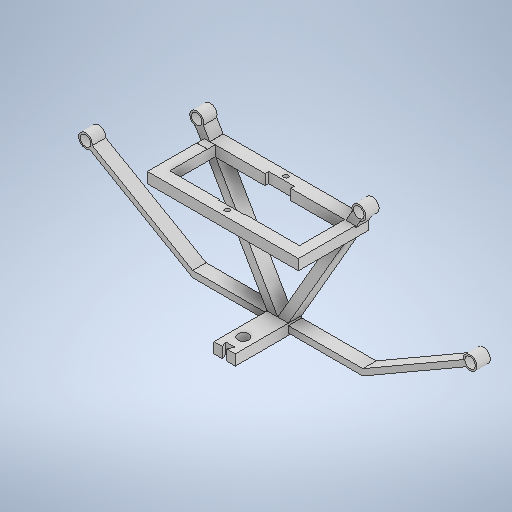
# Autodesk Inventor part: pelvis øvre del stor servo
Saved by Autodesk Inventor 2025.1 (Build 291241020, 241B)
## iProperties
Created: 2025-01-28
Part Number: pelvis øvre del stor servo
Material: Generic
Document SubType Name: Modeling
Designer: morte
Density: 1 g/cm^3
Appearance: Default
Author: morte
Autodesk Inventor part; units mm, degrees
ref_plane "XZ Plane" through (0, 0, 0) normal (0, 1, 0) x (-1, 0, 0)
ref_plane "XY Plane" through (0, 0, 0) normal (0, 0, 1) x (1, 0, 0)
sketch "Sketch1" plane through (0, 0, 0) normal (0, 0, 1) x (1, 0, 0)
  line L0 (5, -2.5) -> (-5, -2.5)
  line L1 (-5, -2.5) -> (-5, 2.5)
  line L2 (-5, 2.5) -> (5, 2.5)
  line L3 (5, 2.5) -> (5, -2.5)
  line L4 (5, -2.5) -> (-5, 2.5) construction
  line L5 (-5, -2.5) -> (5, 2.5) construction
  point P0 (0, 0)
  dimension "d0" = 10
  dimension "d1" = 5
  constraints: 12 end point, 2 midpoint, 2 parallel, 1 horizontal, 1 perpendicular
  measures "d0" distance of L1.end L2.end
  measures "d1" distance of L0.end L1.end
extrude "Extrusion1" add sketch "Sketch1" against normal blind 30
sketch "Sketch2" plane through (0, 0, 0) normal (0, 1, 0) x (-1, 0, 0)
  line L0 (0, 0) -> (0, -2.65)
  line L1 (0, -2.65) -> (2.075, -2.65)
  line L2 (0, -2.65) -> (-2.075, -2.65)
  line L3 (0, 0) -> (-1.075, 0)
  line L4 (-5, 0) -> (5, 0) projected
  line L5 (0, 0) -> (1.075, 0)
  line L6 (2.075, -2.65) -> (1.075, 0)
  line L7 (-2.075, -2.65) -> (-1.075, 0)
  point P0 (-0.025, -2.7)
  dimension "d13" = 2.075
  dimension "d74" = 2.075
  dimension "d75" = 1.075
  dimension "d76" = 1.075
  dimension "d77" = 2.65
  constraints: 14 end point, 2 point on line, 1 horizontal, 1 midpoint, 1 perpendicular, 1 vertical
  measures "d13" distance of L0.end L1.end
  measures "d74" distance of L0.end L2.end
  measures "d75" distance of L0.start L3.end
  measures "d76" distance of L0.start L5.end
  measures "d77" distance of point (0, 0) L0.end
extrude "Extrusion2" cut sketch "Sketch2" along normal through all both and the other way through all
sketch "Sketch3" plane through (0, 0, -30) normal (0, 0, -1) x (-1, 0, 0)
  line L0 (5, -2.5) -> (5, 2.5) projected
  line L1 (5, 0) -> (5, 1.5)
  line L2 (5, 1.5) -> (40, 1.5)
  line L3 (5, 1.5) -> (40, 1.5) construction
  line L4 (40, 1.5) -> (40, -1.5)
  line L5 (40, -1.5) -> (5, -1.5)
  line L6 (5, 1.5) -> (5, -1.5)
  line L7 (-5, 2.5) -> (-5, -2.5) projected
  line L8 (-5, -1.5) -> (-5, 1.5)
  line L9 (-5, 0) -> (-5, 1.5)
  line L10 (-5, 0) -> (-5, -1.5)
  line L11 (-40, -1.5) -> (-40, 1.5004)
  line L12 (-40, 1.5004) -> (-5, 1.5)
  line L13 (-5, 0) -> (-5, -1.5)
  line L14 (-5, -1.5) -> (-40, -1.5)
  point P0 (0, 0)
  point P1 (5, 0)
  dimension "d17" = 35
  dimension "d19" = 3
  dimension "d26" = 1.5
  dimension "d28" = 1.5
  dimension "d29" = 35
  dimension "d30" = 35
  dimension "d31" = 1.5
  constraints: 26 end point, 6 point on line, 5 midpoint, 4 collinear, 3 perpendicular, 2 horizontal
  measures "d17" distance of L1.end L2.end
  measures "d19" distance of L2.end L4.end
  measures "d26" distance from line of point (-5, 0) L12
  measures "d28" distance of L13.start L13.end
  measures "d29" distance of L11.end L8.end
  measures "d30" distance of L13.end L11.start
  measures "d31" distance from line of point (5, 0) L2
extrude "Extrusion3" add sketch "Sketch3" against normal blind 5
sketch "Sketch4" plane through (0, 0, -30) normal (0, 0, -1) x (-1, 0, 0)
  line L0 (40, -1.5) -> (40, 1.5) projected
  line L1 (40, -1.5) -> (97.5, -1.5) construction
  line L2 (40, 1.5) -> (5, 1.5) projected
  line L3 (40, 1.5) -> (87.6314, 29)
  line L4 (40, 1.5) -> (95, 1.5) construction
  line L5 (5, -1.5) -> (40, -1.5) projected
  line L6 (40, -1.5) -> (88.9304, 26.75)
  line L7 (88.9304, 26.75) -> (87.6314, 29)
  line L8 (-5, -1.5) -> (-40, -1.5) projected
  line L9 (-40, -1.5) -> (-88.9306, 26.7501)
  line L10 (-40, -1.5) -> (18, -1.5) construction
  line L11 (-40, 1.5004) -> (-5, 1.5) projected
  line L12 (-40, 1.5004) -> (-87.6314, 29.0004)
  line L13 (-40, 1.5004) -> (15, 1.5004) construction
  line L14 (-87.6314, 29.0004) -> (-88.9306, 26.7501)
  line L15 (87.6314, 29) -> (88.2809, 27.875)
  line L16 (88.2809, 27.875) -> (90.446, 29.125)
  line L17 (88.2809, 27.875) -> (90.7809, 27.875) construction
  circle A0 centre (90.446, 29.125) radius 2.5
  arc A1 (88.5627, 26.5377) -> (87.2514, 28.7806) centre (90.4788, 29.1627) ccw
  line L18 (-88.281, 27.8752) -> (-90.4461, 29.1252)
  line L19 (-88.281, 27.8752) -> (-85.781, 27.8752) construction
  circle A2 centre (-90.4461, 29.1252) radius 2.5
  arc A3 (-87.1694, 28.7337) -> (-88.4686, 26.4834) centre (-90.4461, 29.1252) ccw
  line L20 (5, 2.5) -> (-5, 2.5) projected
  line L21 (0, 2.5) -> (-35, 63.1218)
  line L22 (0, 2.5) -> (70, 2.5) construction
  line L23 (0, 2.5) -> (35, 63.1218)
  line L24 (0, 2.5) -> (70, 2.5) construction
  line L25 (-5, 2.5) -> (-38.75, 60.9567)
  line L26 (-5, 2.5) -> (68.5, 2.5) construction
  line L27 (5, 2.5) -> (38.75, 60.9567)
  line L28 (5, 2.5) -> (73.5, 2.5) construction
  line L29 (-35, 63.1218) -> (-38.75, 60.9567)
  line L30 (35, 63.1218) -> (38.75, 60.9567)
  line L31 (-36.875, 62.0392) -> (-38.125, 64.2043)
  circle A4 centre (-38.125, 64.2043) radius 2.5
  line L32 (36.875, 62.0392) -> (38.125, 64.2043)
  circle A5 centre (38.125, 64.2043) radius 2.5
  line L33 (-40, -1.5) -> (-40, 1.5004) projected
  line L34 (-40, 1.5004) -> (-40, -1.5)
  line L35 (40, 1.5) -> (40, -1.5)
  line L36 (-5, 2.5) -> (-5, 1.5) projected
  line L37 (-5, 2.5) -> (0, 2.5)
  line L38 (0, 2.5) -> (5, 2.5)
  arc A6 (38.75, 60.9567) -> (35, 63.1218) centre (38.125, 64.2043) ccw
  arc A7 (-35, 63.1218) -> (-38.75, 60.9567) centre (-38.125, 64.2043) ccw
  point P0 (0, 0)
  dimension "d58" = 5
  dimension "d34" = 55
  dimension "d35" = 30
  dimension "d38" = 150
  dimension "d39" = 55
  dimension "d40" = 150
  dimension "d41" = 2.5
  dimension "d42" = 30
  dimension "d43" = 0.8
  dimension "d44" = 2.5
  dimension "d45" = 150
  dimension "d46" = 0.8
  dimension "d47" = 120
  dimension "d48" = 60
  dimension "d49" = 70
  dimension "d50" = 70
  dimension "d52" = 120
  dimension "d54" = 60
  dimension "d55" = 2.5
  dimension "d59" = 2.5
  constraints: 62 end point, 10 horizontal, 8 point on circle, 7 coincident, 6 equal length, 6 perpendicular, 5 midpoint, 4 centre point, 4 point on line, 3 collinear, 12 other
  measures "d34" distance of L0.end L3.end
  measures "d35" angle of L4 L3
  measures "d38" angle of L10 L9
  measures "d39" distance of L11.start L12.end
  measures "d40" angle of L13 L12
  measures "d41" distance of L15.end L16.end
  measures "d42" angle of L17 L16
  measures "d44" distance of L18.start L18.end
  measures "d45" angle of L19 L18
  measures "d47" angle of L22 L21
  measures "d48" angle of L24 L23
  measures "d49" distance of L21.end L21.start
  measures "d50" distance of L21.start L23.end
  measures "d52" angle of L26 L25
  measures "d54" angle of L28 L27
  measures "d55" distance of L31.start L31.end
  measures "d59" distance of L32.start L32.end
extrude "Extrusion4" add sketch "Sketch4" against normal blind 5
sketch "Sketch5" plane through (-5, -2.5, -30) normal (0, -1, 0) x (1, 0, 0)
  line L0 (0, 5) -> (0, 0) projected
  line L1 (0, 0) -> (0, 21.2)
  line L2 (0, 30) -> (0, 5) projected
  line L3 (0, 21.2) -> (1.9, 21.2) construction
  line L4 (0, 21.2) -> (1.9, 21.2) construction
  line L5 (1.9, 21.2) -> (5, 21.2)
  line L6 (2.95, 23.25) -> (7.05, 19.15) construction
  line L7 (7.05, 23.25) -> (2.95, 19.15) construction
  circle A0 centre (5, 21.2) radius 2.6
  line L8 (5, 21.2) -> (0, 21.2)
  point P0 (5, 30)
  dimension "d64" = 21.2
  dimension "d66" = 0
  dimension "d69" = 4.1
  dimension "d70" = 4.1
  dimension "d78" = 5.2
  dimension "d79" = 5
  constraints: 14 end point, 3 horizontal, 2 collinear, 2 midpoint, 1 centre point, 1 coincident, 1 point on line
  measures "d64" distance of L0.end L1.end
  measures "d66" distance between parallel lines of L3 L4
  measures "d69" distance of L6.end L7.end
  measures "d70" distance of L7.start L6.end
  measures "d78" diameter of A0
  measures "d79" distance of L1.end L5.end
extrude "Extrusion5" cut sketch "Sketch5" against normal through all
ref_plane "Work Plane1" through (-32, 0, 0) normal (1, 0, 0) x (0, 1, 0)
sketch "Sketch6" plane through (-32, 0, 0) normal (1, 0, 0) x (0, 1, 0)
  line L0 (0, 0) -> (0, -25)
  line L1 (-1.5, -25) -> (1.5, -25) projected
  line L2 (0, -25) -> (49.2334, -25)
  line L3 (63.1218, -25) -> (2.5, -25) projected
  line L4 (49.2334, -25) -> (49.2334, -21.4137)
  line L5 (49.2334, -21.4137) -> (57.9156, -21.4137)
  line L6 (57.9156, -21.4137) -> (57.9156, -25)
  constraints: 10 end point, 2 perpendicular, 2 point on line, 1 midpoint, 1 vertical
extrude "Extrusion6" add sketch "Sketch6" along normal mid plane 5
sketch "Sketch7" plane through (-31.9816, 49.2334, -25) normal (0, 0, -1) x (-1, 0, 0)
  line L0 (2.5184, 8.6821) -> (-2.4816, 8.6821) projected
  line L1 (-2.4816, 0) -> (2.5184, 0) projected
  line L2 (2.5184, 8.6821) -> (2.5184, 0)
  line L3 (2.5184, 0) -> (-2.4816, 0)
  line L4 (-2.4816, 0) -> (-2.4816, 8.6821)
  line L5 (-2.4816, 8.6821) -> (2.5184, 8.6821)
  point P0 (-31.9816, -49.2334)
  dimension "d125" = 8.6821
  constraints: 8 end point, 3 perpendicular, 1 vertical
  measures "d125" distance of L1.start L4.end
extrude "Extrusion7" add sketch "Sketch7" along normal blind 5
sketch "Sketch8" plane through (-34.5, 49.2334, -21.4137) normal (0, 0, 1) x (1, 0, 0)
  line L0 (2.5184, 0) -> (0, 0) projected
  line L1 (5, 4.3621) -> (5, 0) projected
  line L2 (0, 0) -> (5, 0)
  line L3 (5, 0) -> (5, 8.7557)
  line L4 (5, 8.7557) -> (0, 8.7557)
  line L5 (0, 0) -> (0, 4.3621) projected
  line L6 (0, 8.7557) -> (0, 0)
  point P0 (34.5, -49.2334)
  constraints: 8 end point, 2 perpendicular, 1 collinear, 1 horizontal
extrude "Extrusion8" add sketch "Sketch8" along normal blind 23.214
sketch "Sketch10" plane through (-29.5, 0, 0) normal (1, 0, 0) x (0, 0, -1)
  line L0 (25, 49.2334) -> (-1.8003, 49.2334) projected
  line L1 (-1.8003, 49.2334) -> (-1.8003, 57.9891) projected
  line L2 (-1.8003, 49.2334) -> (-1.8003, 57.9891)
  line L3 (-1.8003, 57.9891) -> (3.6997, 57.9891)
  line L4 (21.4137, 57.9891) -> (-1.8003, 57.9891) projected
  line L5 (3.6997, 57.9891) -> (3.6997, 49.2334)
  line L6 (3.6997, 49.2334) -> (-1.8003, 49.2334)
  line L7 (-1.8003, 57.9891) -> (-1.8003, 49.2334)
  point P0 (0, 0)
  dimension "d87" = 5.5
  constraints: 10 end point, 2 perpendicular, 1 collinear, 1 point on line, 1 vertical
  measures "d87" distance of L1.end L3.end
extrude "Extrusion9" add sketch "Sketch10" along normal blind 66
sketch "Sketch11" plane through (-29.5, 49.2334, -3.6997) normal (0, 0, -1) x (-1, 0, 0)
  line L0 (5, 0) -> (-66, 0) projected
  line L1 (-66, 8.7557) -> (-66, 0) projected
  line L2 (-66, 0) -> (-66, 8.7557)
  line L3 (-66, 8.7557) -> (-61, 8.7557)
  line L4 (-61, 8.7557) -> (-61, 0)
  line L5 (-61, 0) -> (-66, 0)
  point P0 (-29.5, -49.2334)
  point P1 (-61, 0)
  dimension "d90" = 5
  dimension "d124" = 8.7557
  constraints: 8 end point, 3 perpendicular, 1 collinear
  measures "d90" distance of L1.start L3.end
  measures "d124" distance of L3.end L4.end
extrude "Extrusion10" add sketch "Sketch11" along normal up to surface (21.3003 mm away)
sketch "Sketch12" plane through (36.5, 49.2334, -25) normal (0, 0, -1) x (-1, 0, 0)
  line L0 (71, 8.7557) -> (0, 8.7557) projected
  line L1 (71, 0) -> (0, 0) projected
  line L2 (0, 8.7557) -> (0, 0) projected
  line L3 (0, 0) -> (0, 8.7557)
  line L4 (0, 8.7557) -> (5, 8.7557)
  line L5 (5, 8.7557) -> (5, 0)
  line L6 (0, 0) -> (5, 0)
  point P0 (36.5, -49.2334)
  dimension "d94" = 5
  constraints: 8 end point, 2 collinear, 2 point on line, 1 perpendicular
  measures "d94" distance of L0.end L4.end
extrude "Extrusion11" add sketch "Sketch12" along normal up to surface (5 mm away)
sketch "Sketch13" plane through (-34.5, 57.9891, -21.4137) normal (0, 1, 0) x (1, 0, 0)
  line L0 (0, -23.214) -> (71, -23.214) projected
  line L1 (34.4572, -23.214) -> (37.4572, -23.214) construction
  line L2 (34.5022, -23.214) -> (34.5022, -20.214)
  line L3 (34.5022, -23.214) -> (37.5022, -23.214) construction
  circle A0 centre (34.5022, -20.214) radius 1.1
  dimension "d100" = 3
  dimension "d101" = 90
  dimension "d102" = 2.2
  constraints: 6 end point, 2 horizontal, 2 perpendicular, 2 point on line, 1 centre point, 1 coincident
  measures "d100" distance of L2.start L2.end
  measures "d101" angle of L3 L2
  measures "d102" diameter of A0
extrude "Extrusion12" cut sketch "Sketch13" against normal blind 11
sketch "Sketch14" plane through (-34.5, 57.9891, -21.4137) normal (0, 1, 0) x (1, 0, 0)
  circle A0 centre (34.5022, -20.214) radius 1.1 projected
  line L0 (34.5022, -20.214) -> (59.5022, -20.214) construction
  line L1 (34.5022, 5.886) -> (34.5022, 7.286)
  line L2 (5, 8.5863) -> (34.5, 8.5863) projected
  line L3 (34.5022, 5.886) -> (35.9022, 5.886) construction
  line L4 (66.5367, 3.5863) -> (71, 3.5863) projected
  line L5 (71, 7.286) -> (71, 3.5863)
  line L6 (0, 7.286) -> (0, 3.5863)
  line L7 (29.5, 3.5863) -> (-5.5, 3.5863) projected
  line L8 (34.5022, 3.686) -> (34.5022, 2.286)
  line L9 (34.5022, 3.686) -> (35.9022, 3.686) construction
  line L10 (34.5, 3.5863) -> (34.5, 8.5863) projected
  line L11 (66.5367, 8.5863) -> (66.5367, 3.5863) projected
  line L12 (2.5058, 3.5863) -> (2.5058, 8.5863) projected
  line L13 (66.5367, 3.5863) -> (2.5058, 3.5863)
  line L14 (2.5058, 3.5863) -> (2.5058, 8.5863)
  line L15 (29.5, 8.5863) -> (-5.5, 8.5863) projected
  line L16 (2.5058, 8.5863) -> (66.5367, 8.5863)
  line L17 (66.5367, 8.5863) -> (66.5367, 3.5863)
  point P0 (34.5, -21.4137)
  dimension "d108" = 1.4
  dimension "d109" = 90
  dimension "d111" = 1.4
  dimension "d112" = 90
  constraints: 22 end point, 5 perpendicular, 3 horizontal, 3 point on line, 1 collinear
  measures "d108" distance of L1.start L1.end
  measures "d109" angle of L3 L1
  measures "d111" distance of L8.start L8.end
  measures "d112" angle of L8 L9
extrude "Extrusion13" add sketch "Sketch14" against normal blind 5 contours L2 L10 L13 L7 L12 L15 | L16 L11 L13 L10
sketch "Sketch15" plane through (0, 0, -30) normal (0, 0, -1) x (-1, 0, 0)
  line L0 (0, 0) -> (0, -2.5)
  line L1 (-2.075, -2.5) -> (2.075, -2.5) projected
  line L2 (5, -2.5) -> (1.075, -2.5) projected
  line L3 (0, -2.5) -> (5, -2.5)
  line L4 (5, -2.5) -> (5, -1.5)
  line L5 (88.5627, 26.5377) -> (40, -1.5) projected
  line L6 (5, -1.5) -> (40, -1.5)
  line L7 (40, -1.5) -> (88.5627, 26.5377)
  line L8 (40, 1.5) -> (87.2514, 28.7806) projected
  line L9 (87.2514, 28.7806) -> (40, 1.5)
  line L10 (5, 1.5) -> (40, 1.5) projected
  line L11 (40, 1.5) -> (5, 1.5)
  line L12 (0, 2.5) -> (5, 2.5) projected
  line L13 (5, 1.5) -> (5, 2.5)
  line L14 (38.75, 60.9567) -> (34.5, 53.5955) projected
  line L15 (5, 2.5) -> (38.75, 60.9567)
  circle A0 centre (38.125, 64.2043) radius 2.5 projected
  arc A1 (38.75, 60.9567) -> (35, 63.1218) centre (38.125, 64.2043) ccw
  circle A2 centre (38.125, 64.2043) radius 2.5
  line L16 (35, 63.1218) -> (0, 2.5)
  line L17 (31.9942, 57.9156) -> (35, 63.1218) projected
  line L18 (-31.5, 57.0596) -> (0, 2.5) projected
  arc A3 (-35, 63.1218) -> (-38.75, 60.9567) centre (-38.125, 64.2043) ccw projected
  line L19 (0, 2.5) -> (-35, 63.1218)
  arc A4 (-35, 63.1218) -> (-38.75, 60.9567) centre (-38.125, 64.2043) ccw
  circle A5 centre (-38.125, 64.2043) radius 2.5
  line L20 (-5, 2.5) -> (-31.9816, 49.2334) projected
  line L21 (-38.75, 60.9567) -> (-5, 2.5)
  line L22 (-5, 2.5) -> (-5, 1.5)
  line L23 (-5, -2.5) -> (-5, 2.5) projected
  line L24 (-40, 1.5004) -> (-5, 1.5) projected
  line L25 (-5, 1.5) -> (-40, 1.5004)
  line L26 (-87.1694, 28.7337) -> (-40, 1.5004) projected
  line L27 (-40, 1.5004) -> (-87.1694, 28.7337)
  circle A6 centre (-90.4461, 29.1252) radius 2.5 projected
  circle A7 centre (-90.4461, 29.1252) radius 2.5
  line L28 (-40, -1.5) -> (-88.4686, 26.4834) projected
  arc A8 (-87.1694, 28.7337) -> (-88.4686, 26.4834) centre (-90.4461, 29.1252) ccw
  line L29 (-88.4686, 26.4834) -> (-40, -1.5)
  line L30 (-5, -1.5) -> (-40, -1.5) projected
  line L31 (-40, -1.5) -> (-5, -1.5)
  line L32 (-5, -1.5) -> (-5, -2.5)
  line L33 (-5, -2.5) -> (5, -2.5)
  line L34 (-5, 1.5) -> (5, 1.5)
  line L35 (-5, -1.5) -> (-5, 1.5) projected
  line L36 (-5, -1.5) -> (-5, 1.5)
  line L37 (5, -1.5) -> (5, 2.5)
  line L38 (40, -1.5) -> (88.5627, 26.5377)
  circle A9 centre (90.446, 29.125) radius 2.5 projected
  arc A10 (88.5627, 26.5377) -> (87.2514, 28.7806) centre (90.4788, 29.1627) ccw projected
  arc A11 (88.5627, 26.5377) -> (87.2514, 28.7806) centre (90.4788, 29.1627) ccw
  circle A12 centre (90.446, 29.125) radius 2.5
  dimension "d117" = 1
  constraints: 50 end point, 14 collinear, 8 centre point, 8 coincident, 8 point on circle, 3 horizontal, 2 concentric, 2 perpendicular, 1 midpoint, 1 point on line
  measures "d117" distance of L2.start L4.end
extrude "Extrusion14" add sketch "Sketch15" along normal blind 1.3
sketch "Sketch17" plane through (0, 0, -30) normal (0, 0, -1) x (-1, 0, 0)
  line L0 (34.5, 49.2334) -> (-36.5, 49.2334) projected
  line L1 (34.5, 49.2334) -> (34.5, 53.5961)
  line L2 (34.5, 53.5961) -> (31.9807, 49.2334)
  point P0 (0, 0)
  constraints: 4 end point, 1 perpendicular, 1 point on line
extrude "Extrusion16" add sketch "Sketch17" along normal blind 1.3
sketch "Sketch18" plane through (36.5, 0, 0) normal (1, 0, 0) x (0, 0, -1)
  line L0 (30, 57.9891) -> (25, 57.9891) projected
  line L1 (25, 57.9891) -> (25, 52.9891)
  line L2 (25, 52.9891) -> (-2.8863, 52.9891)
  line L3 (-2.8863, 52.9891) -> (-2.8863, 45.156)
  line L4 (-2.8863, 45.156) -> (25, 45.156)
  line L5 (25, 2.5) -> (25, 49.2334) projected
  line L6 (25, 52.9891) -> (25, 45.156)
  line L7 (25, 57.9891) -> (25, 49.2334) projected
  point P0 (0, 0)
  point P1 (31.2997, 57.9891)
  point P2 (25, 57.0596)
  point P3 (31.3, 57.9891)
  dimension "d126" = 5
  constraints: 10 end point, 2 perpendicular, 1 collinear, 1 horizontal, 1 point on line, 1 vertical
  measures "d126" distance of L0.end L1.end
extrude "Extrusion17" cut sketch "Sketch18" against normal through all
sketch "Sketch20" plane through (0, 0, -30) normal (0, 0, -1) x (-1, 0, 0)
  line L0 (34.5, 57.9891) -> (-36.5, 57.9891) projected
  line L1 (29.1499, 52.9891) -> (31.9942, 57.9156) projected
  line L2 (32.0367, 57.9891) -> (29.1499, 52.9891)
  line L3 (-32.0367, 57.9891) -> (-29.1499, 52.9891) projected
  line L4 (29.1499, 52.9891) -> (-29.1499, 52.9891)
  line L5 (-29.1499, 52.9891) -> (-32.0367, 57.9891)
  line L6 (-32.0367, 57.9891) -> (32.0367, 57.9891)
  point P0 (0, 0)
  constraints: 8 end point, 2 collinear, 1 horizontal, 1 parallel, 1 point on line
extrude "Extrusion18" add sketch "Sketch20" along normal blind 1.3
sketch "Sketch21" plane through (-34.5, 57.9891, -21.4137) normal (0, 1, 0) x (1, 0, 0)
  circle A0 centre (34.5022, -20.214) radius 1.1 projected
  circle A1 centre (34.5, 7.386) radius 1.1
  point P0 (34.5, -21.4137)
  dimension "d133" = 2.2
  constraints: 1 centre point
  measures "d133" diameter of A1
extrude "Extrusion19" cut sketch "Sketch21" against normal blind 10 contours A1
sketch "Sketch22" plane through (-34.5, 57.9891, -21.4137) normal (0, 1, 0) x (1, 0, 0)
  circle A0 centre (34.5022, -20.214) radius 1.1 projected
  line L0 (34.5022, -19.114) -> (34.5022, -18.114)
  line L1 (66, -17.714) -> (5, -17.714) projected
  line L2 (34.5022, -19.114) -> (35.5022, -19.114) construction
  line L3 (34.5022, -18.114) -> (28.5021, -18.114)
  line L4 (5, -18.114) -> (5, -17.714)
  line L5 (5, -17.714) -> (66, -17.714)
  line L6 (66, -17.714) -> (66, -17.914)
  line L7 (40.5021, -18.0759) -> (34.5022, -18.114)
  line L8 (34.5022, -18.114) -> (40.5021, -18.0759)
  line L9 (40.5021, -18.0759) -> (40.5021, -17.714)
  line L10 (40.5021, -17.714) -> (28.5021, -17.714)
  line L11 (28.5021, -17.714) -> (28.5021, -18.114)
  point P0 (34.5, -21.4137)
  dimension "d136" = 1
  dimension "d137" = 90
  dimension "d149" = 6
  dimension "d150" = 12
  constraints: 22 end point, 5 perpendicular, 2 point on line, 1 collinear, 1 horizontal, 1 parallel, 1 vertical, 1 vertical alignment, 1 other
  measures "d136" distance of L0.start L0.end
  measures "d137" angle of L2 L0
  measures "d149" distance of L7.start L0.end
  measures "d150" distance of L9.end L10.end
extrude "Extrusion20" cut sketch "Sketch22" against normal blind 10 contours L3 L11 L1 L9 L7
sketch "Sketch25" plane through (-34.5, 57.9891, -21.4137) normal (0, 1, 0) x (1, 0, 0)
  circle A0 centre (34.5, 7.386) radius 1.1 projected
  line L0 (34.5, 6.286) -> (34.5, 5.286)
  line L1 (34.5, 3.5863) -> (34.5, 9.8863) projected
  line L2 (34.5, 5.286) -> (40.5, 5.286)
  line L3 (40.5, 5.286) -> (40.5, 3.5863)
  line L4 (63.6499, 3.5863) -> (5.3501, 3.5863) projected
  line L5 (40.5, 3.5863) -> (28.5, 3.5863)
  line L6 (28.5, 3.5863) -> (28.5, 5.286)
  line L7 (28.5, 5.286) -> (34.5, 5.286)
  point P0 (34.5, -21.4137)
  dimension "d144" = 1
  dimension "d145" = 6
  dimension "d146" = 12
  constraints: 12 end point, 4 perpendicular, 4 point on line, 1 vertical alignment, 1 other
  measures "d144" distance of L0.start L0.end
  measures "d145" distance of L0.end L2.end
  measures "d146" distance of L3.end L5.end
extrude "Extrusion21" cut sketch "Sketch25" against normal blind 10 contours L2 L3 L4 L1 | L1 L4 L6 L7
sketch "Sketch26" plane through (0, 0, -25) normal (0, 0, 1) x (1, 0, 0)
  line L0 (-5, 2.5) -> (-31.9816, 49.2334) projected
  line L1 (-34.5, 49.2334) -> (-34.5, 53.5955) projected
  line L2 (-31.9816, 49.2334) -> (-34.5, 53.5955)
  line L3 (-31.9816, 49.2334) -> (-34.5, 49.2334) projected
  line L4 (-34.5, 53.5955) -> (-34.5, 49.2334)
  line L5 (-34.5, 49.2334) -> (-31.9816, 49.2334)
  point P0 (0, 0)
  constraints: 6 end point, 2 perpendicular
extrude "Extrusion22" cut sketch "Sketch26" against normal blind 10
sketch "Sketch27" plane through (0, 0, -25) normal (0, 0, 1) x (1, 0, 0)
  line L0 (31.9816, 49.2334) -> (36.5, 49.2334) projected
  line L1 (36.5, 57.0596) -> (38.75, 60.9567) projected
  line L2 (31.9816, 49.2334) -> (36.5, 57.0596)
  line L3 (36.5, 57.0596) -> (36.5, 49.2334)
  line L4 (36.5, 49.2334) -> (31.9816, 49.2334)
  point P0 (0, 0)
  constraints: 6 end point, 1 collinear, 1 perpendicular
extrude "Extrusion23" cut sketch "Sketch27" against normal blind 10
sketch "Sketch28" plane through (0, 0, -25) normal (0, 0, -1) x (-1, 0, 0)
  line L0 (-36.5, 57.9891) -> (-36.5, 52.9891) projected
  line L1 (-36.5, 52.9891) -> (-34.1499, 52.9891) projected
  line L2 (-36.5, 52.9891) -> (-34.1499, 52.9891)
  line L3 (-36.5, 57.0596) -> (-34.1499, 52.9891) projected
  line L4 (-34.1499, 52.9891) -> (-36.5, 57.0596)
  line L5 (-36.5, 57.0596) -> (-36.5, 52.9891)
  point P0 (0, 0)
  constraints: 6 end point, 2 collinear, 1 perpendicular
extrude "Extrusion24" add sketch "Sketch28" along normal up to surface (6.3 mm away)
body "Solid1"
